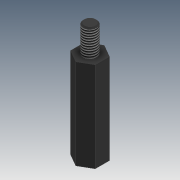
# Autodesk Inventor part: 20mm_support
Saved by Autodesk Inventor 2020 (Build 240168000, 168)
## iProperties
Created: 2020-09-27
Part Number: 20mm_support
Material: Generic
Document SubType Name: Modeling
Designer: DELL
Density: 1 g/cm^3
Appearance: Rubber - Black
Author: DELL
Autodesk Inventor part; units mm, degrees
ref_plane "YZ Plane" through (0, 0, 0) normal (1, 0, 0) x (0, 1, 0)
ref_plane "XZ Plane" through (0, 0, 0) normal (0, 1, 0) x (-1, 0, 0)
ref_plane "XY Plane" through (0, 0, 0) normal (0, 0, 1) x (1, 0, 0)
sketch "Sketch1" plane through (0, 0, 0) normal (0, 1, 0) x (-1, 0, 0)
  line L0 (0, 3.1639) -> (2.74, 1.5819)
  line L1 (2.74, 1.5819) -> (2.74, -1.5819)
  line L2 (2.74, -1.5819) -> (0, -3.1639)
  line L3 (0, -3.1639) -> (-2.74, -1.5819)
  line L4 (-2.74, -1.5819) -> (-2.74, 1.5819)
  line L5 (-2.74, 1.5819) -> (0, 3.1639)
  point P0 (0, 0)
  point P1 (0, 0)
  dimension "d0" = 5.48
  constraints: 12 end point, 1 coincident, 1 vertical, 13 other
  measures "d0" distance between parallel lines of L4 L1
extrude "Extrusion1" add sketch "Sketch1" along normal blind 20
sketch "Sketch2" plane through (0, 20, 0) normal (0, 1, 0) x (1, 0, 0)
  circle A0 centre (0, 0) radius 1.5
  dimension "d3" = 3
  constraints: 1 centre point, 1 coincident
  measures "d3" diameter of A0
extrude "Extrusion2" add sketch "Sketch2" along normal blind 6
thread "Thread1" size "M3x0.5" class "6g" standard "ANSI Metric M Profile" full length
chamfer "Chamfer1" distance 0.3 angle 45 1 edges at (-1.5, 26, 0)
sketch "Sketch3" plane through (0, 0, 0) normal (0, -1, 0) x (1, 0, 0)
  circle A0 centre (0, 0) radius 1.5
  dimension "d11" = 3
  constraints: 1 centre point, 1 coincident
  measures "d11" diameter of A0
extrude "Extrusion3" cut sketch "Sketch3" against normal blind 7
thread "Thread2" size "M3x0.5" class "6H" standard "ANSI Metric M Profile" full length
chamfer "Chamfer2" distance 0.3 angle 45 1 edges at (-1.5, 0, 0)
body "Solid1"
